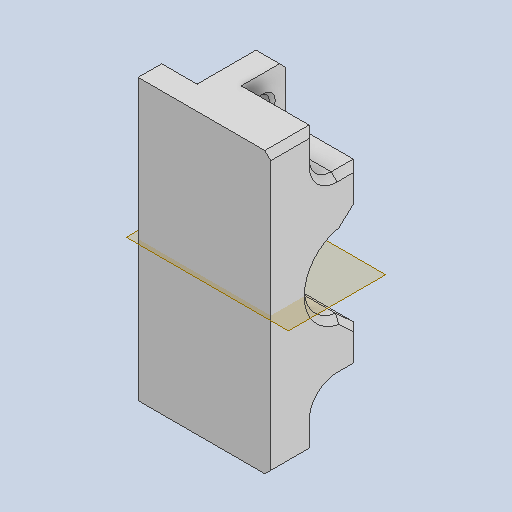
# Autodesk Inventor part: pillar_placer
Saved by Autodesk Inventor 2024 (Build 280153000, 153)
## iProperties
Created: 2021-06-14
Part Number: pillar_placer
Material: Generic
Document SubType Name: Modeling
Designer: dsdan
Density: 1 g/cm^3
Appearance: Default
Author: dsdan
Autodesk Inventor part; units mm, degrees
ref_plane "YZ Plane" through (0, 0, 0) normal (1, 0, 0) x (0, 1, 0)
ref_plane "XZ Plane" through (0, 0, 0) normal (0, 1, 0) x (-1, 0, 0)
ref_plane "XY Plane" through (0, 0, 0) normal (0, 0, 1) x (1, 0, 0)
sketch "Sketch1" plane through (0, 0, 0) normal (0, 0, 1) x (1, 0, 0)
  line L0 (0, 0) -> (45, 0)
  line L1 (45, 0) -> (45, -95)
  line L2 (45, -95) -> (0, -95)
  line L3 (0, -95) -> (0, 0)
  dimension "d14" = 95
  dimension "d15" = 45
  constraints: 8 end point, 2 parallel, 1 horizontal, 1 perpendicular
  measures "d14" distance of L0.end L1.end
  measures "d15" distance between parallel lines of L3 L1
extrude "Extrusion1" add sketch "Sketch1" against normal blind 30
sketch "Sketch2" plane through (0, 0, -30) normal (0, 0, -1) x (-1, 0, 0)
  line L0 (0, -95) -> (0, 0) projected
  line L1 (0, 0) -> (-12, 0)
  line L2 (-12, 0) -> (-12, -95)
  line L3 (-12, -95) -> (0, -95)
  line L4 (0, -95) -> (0, 0)
  line L5 (-45, -95) -> (0, -95) projected
  dimension "d2" = 12
  constraints: 8 end point, 2 parallel, 1 collinear, 1 horizontal, 1 perpendicular
  measures "d2" distance between parallel lines of L0 L2
extrude "Extrusion2" cut sketch "Sketch2" against normal blind 20
sketch "Sketch3" plane through (45, -95, 0) normal (1, 0, 0) x (0, 0, -1)
  circle A0 centre (25.875, 47.5) radius 15.621 construction
  circle A1 centre (25.875, 47.5) radius 12.5
  line L0 (0, 0) -> (0, 95) construction
  line L1 (0, 0) -> (30, 0) projected
  line L2 (30, 0) -> (0, 95) construction
  line L3 (30, 95) -> (0, 0) construction
  point P0 (15, 47.5)
  point P1 (10, 95)
  dimension "d5" = 31.242
  dimension "d6" = 25
  dimension "d13" = 15.875
  constraints: 4 end point, 2 centre point, 2 coincident, 1 horizontal alignment, 1 midpoint
  measures "d5" diameter of A0
  measures "d6" diameter of A1
  measures "d13" horizontal distance of point (10, 95) A1.centre
extrude "Extrusion3" cut sketch "Sketch3" against normal through all
sketch "Sketch4" plane through (12, 0, -10) normal (-1, 0, 0) x (0, 0, 1)
  arc A0 (-20, -59.2998) -> (-20, -35.7002) centre (-15.875, -47.5) ccw projected
  circle A1 centre (-15.875, -47.5) radius 20
  point P0 (10, 0)
  dimension "d9" = 40
  constraints: 1 centre point, 1 coincident
  measures "d9" diameter of A1
extrude "Extrusion4" cut sketch "Sketch4" against normal blind 13
sketch "Sketch5" plane through (45, -95, 0) normal (1, 0, 0) x (0, 0, -1)
  arc A0 (15, 84.9933) -> (22.5, 77.4933) centre (22.5, 84.9933) ccw
  circle A1 centre (22.5, 84.9933) radius 2.5 construction
  line L0 (22.5, 77.4933) -> (30, 77.4933)
  line L1 (30, 95) -> (30, 59.2998) projected
  line L2 (15, 84.9933) -> (15, 95)
  line L3 (0, 95) -> (30, 95) projected
  point P0 (15.0002, 95)
  dimension "d17" = 15
  constraints: 4 end point, 2 point on circle, 2 tangent, 1 centre point, 1 concentric, 1 horizontal, 1 midpoint, 1 perpendicular, 1 point on line
  measures "d17" diameter of A0
extrude "Extrusion5" cut sketch "Sketch5" against normal blind 25
sketch "Sketch6" plane through (20, -95, 0) normal (1, 0, 0) x (0, 0, -1)
  arc A0 (15, 84.9933) -> (22.5, 77.4933) centre (22.5, 84.9933) ccw projected
  circle A1 centre (22.5, 84.9933) radius 3
  point P0 (0, 95)
  point P1 (15.0002, 95)
  dimension "d20" = 6
  constraints: 1 centre point, 1 coincident
  measures "d20" diameter of A1
extrude "Extrusion6" cut sketch "Sketch6" against normal through all
ref_plane "Work Plane1" through (0, -47.5, 0) normal (0, 1, 0) x (1, 0, 0)
mirror "Mirror1" about plane through (0, -47.5, 0) normal (0, 1, 0) of "Extrusion5", "Extrusion6"
chamfer "Chamfer3" distance 6 angle 45 2 edges at (35, -59.2998, -30) (35, -35.7002, -30)
chamfer "Chamfer1" distance 2 angle 45 20 edges at (45, -5.0033, -15) (45, -15.31, -17.1967) (45, -17.5067, -26.25) (45, -89.9967, -15) (45, -79.69, -17.1967) (45, -77.4933, -26.25) (16, 0, -30) (16, -95, -30) (45, 0, -7.5) (6, 0, -10) (45, -95, -7.5) (6, -95, -10) (45, -23.6034, -30) (45, -47.5, -13.375) (45, -71.3966, -30) (25, -47.5, -13.375) (12, -28.7443, -18.9306) (12, -66.2557, -18.9306) (45, -32.4188, -27.0132) (45, -62.5812, -27.0132)
chamfer "Chamfer2" distance 1 angle 45 2 edges at (20, -10.0067, -19.5) (20, -84.9933, -19.5)
body "Solid1"
